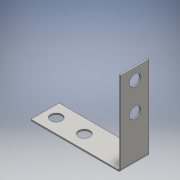
# Autodesk Inventor part: maker-beam-corner
Saved by Autodesk Inventor 2016 (Build 200138000, 138)
## iProperties
Created: 2015-10-07
Part Number: maker-beam-corner
Material: Generic
Document SubType Name: Sheet Metal
Designer: Thomas
Density: 1 g/cm^3
Sheet Metal Rule: Default_mm
Appearance: Default
Author: Thomas
Autodesk Inventor part; units mm, degrees
ref_plane "YZ Plane" through (0, 0, 0) normal (1, 0, 0) x (0, 1, 0)
ref_plane "XZ Plane" through (0, 0, 0) normal (0, 1, 0) x (-1, 0, 0)
ref_plane "XY Plane" through (0, 0, 0) normal (0, 0, 1) x (1, 0, 0)
sketch "Sketch1" plane through (0, 0, 0) normal (0, 0, 1) x (1, 0, 0)
  line L0 (-16, -5) -> (16, -5)
  line L1 (16, -5) -> (16, 5)
  line L2 (16, 5) -> (-16, 5)
  line L3 (-16, 5) -> (-16, -5)
  line L4 (-16, -5) -> (16, 5) construction
  line L5 (16, -5) -> (-16, 5) construction
  point P0 (0, 0)
  dimension "d0" = 32
  dimension "d1" = 10
  measures "d0" distance of L2.end L1.end
  measures "d1" distance of L1.end L0.end
extrude "Plate1" add sketch "Sketch1" along normal blind 0.5
sketch "Sketch2" plane through (15.5, 5, 0) normal (1, 0, 0) x (0, 1, 0)
  line L0 (-10, 0) -> (0, 0)
  line L1 (0, 0) -> (0, 30)
  line L2 (0, 30) -> (-10, 30)
  line L3 (-10, 30) -> (-10, 0)
  constraints: 6 end point, 1 horizontal, 1 perpendicular, 1 vertical
edge flange "Flange1" height 30 angle 90 thickness 0.5 bend radius 0.5 thickness toward (1, 0, 0) relief tear relief width 0.5 relief depth 0.25 edges at (16, 0, 0.5) wall of the first edge with corners at (15.5, -5, 0) (15.5, 5, 0) (15.5, 5, 30) (15.5, -5, 30)
bend "Bend1"
corner "Corner1"
sketch "Sketch4" plane through (0, 0, 0.5) normal (0, 0, 1) x (1, 0, 0)
  line L0 (-16, -5) -> (-16, 5) projected
  point P0 (0, 0)
  point P1 (-12, 0)
  point P2 (-2, 0)
  dimension "d13" = 4
  dimension "d14" = 14
  measures "d13" distance from line of L0 point (-12, 0)
  measures "d14" distance from line of L0 point (-2, 0)
hole "Hole1" at (-12, 0, 0.5) at (-2, 0, 0.5) direction (0, 0, -1) diameter 4 end through all
sketch "Sketch5" plane through (16, -5, 30) normal (1, 0, 0) x (0, 0, -1)
  line L0 (0, 0) -> (0, 10) projected
  point P0 (30, 5)
  point P1 (4, 5)
  point P2 (14, 5)
  dimension "d22" = 4
  dimension "d23" = 14
  measures "d22" distance from line of L0 point (4, 5)
  measures "d23" distance from line of L0 point (14, 5)
hole "Hole2" at (16, 0, 26) at (16, 0, 16) direction (-1, 0, 0) diameter 4 end through all
equation "\"d20\" = Thickness"
equation "\"d29\" = Thickness"
equation "\"d3\" = BendReliefWidth"
equation "\"d4\" = BendReliefDepth"
equation "\"d5\" = MinimumRemnant"
equation "\"d6\" = BendRadius"
equation "\"d9\" = BendRadius"
equation "\"d10\" = CornerReliefSize"
equation "\"d11\" = GapSize"
equation "\"d12\" = JacobiRadiusSize"
equation "\"BendRadius\" = Thickness"
equation "\"BendReliefWidth\" = Thickness"
equation "\"BendReliefDepth\" = 0.5 * Thickness"
equation "\"CornerReliefSize\" = 4 * Thickness"
equation "\"MinimumRemnant\" = 2 * Thickness"
equation "\"TransitionRadius\" = BendRadius"
equation "\"JacobiRadiusSize\" = BendRadius"
equation "\"GapSize\" = Thickness"
equation "\"d2\" = BendRadius"
equation "\"Thickness\" = 0.5"
body "Solid1"
